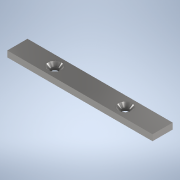
# Autodesk Inventor part: Parte5-Placa
Saved by Autodesk Inventor 2021 (Build 250183000, 183)
## iProperties
Created: 2020-10-13
Part Number: Parte5-Placa
Material: Steel, Carbon
Document SubType Name: Modeling
Designer: oswal
Density: 7.85 g/cm^3
Appearance: Semi-Polished
Author: oswal
Autodesk Inventor part; units mm, degrees
ref_plane "YZ Plane" through (0, 0, 0) normal (1, 0, 0) x (0, 1, 0)
ref_plane "XZ Plane" through (0, 0, 0) normal (0, 1, 0) x (-1, 0, 0)
ref_plane "XY Plane" through (0, 0, 0) normal (0, 0, 1) x (1, 0, 0)
sketch "Sketch1" plane through (0, 0, 0) normal (0, 1, 0) x (-1, 0, 0)
  line L0 (72, -10) -> (-72, -10)
  line L1 (-72, -10) -> (-72, 10)
  line L2 (-72, 10) -> (72, 10)
  line L3 (72, 10) -> (72, -10)
  circle A0 centre (35, 0) radius 3.5
  circle A1 centre (-35, 0) radius 3.5
  point P0 (0, 0)
  dimension "d0" = 144
  dimension "d1" = 20
  dimension "d2" = 72
  dimension "d3" = 10
  dimension "d4" = 35
  dimension "d5" = 35
  dimension "d6" = 7
  dimension "d7" = 70
  constraints: 8 end point, 2 centre point, 2 parallel, 1 equal radius, 1 horizontal, 1 perpendicular
  measures "d0" distance of L1.end L2.end
  measures "d1" distance of L0.end L1.end
  measures "d2" distance from line of L3 point (0, 0)
  measures "d3" distance from line of L2 point (0, 0)
  measures "d4" distance of point (0, 0) A0.centre
  measures "d5" distance of point (0, 0) A1.centre
  measures "d6" diameter of A0
  measures "d7" distance of A1.centre A0.centre
extrude "Extrusion1" add sketch "Sketch1" along normal blind 6
chamfer "Chamfer1" distance 3 angle 45 2 edges at (-31.5, 6, 0) (38.5, 6, 0)
equation "\"d2\" = 0.5 * d0"
equation "\"d3\" = 0.5 * d1"
body "Solid1"
